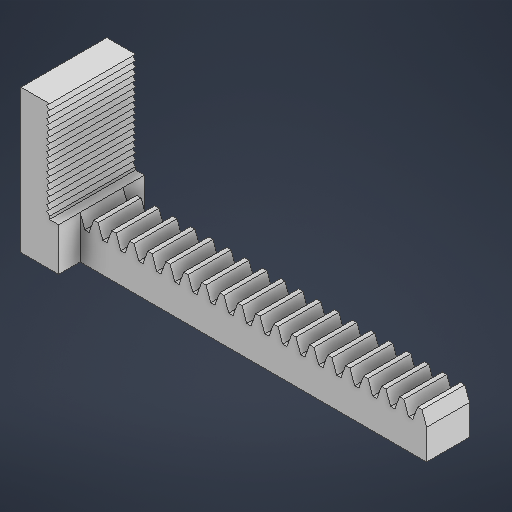
# Autodesk Inventor part: cremallera
Saved by Autodesk Inventor 2025.3 (Build 293356000, 356)
## iProperties
Created: 2024-05-21
Part Number: cremallera
Material: Genérico
Document SubType Name: Modeling
Designer: Jonathan Galarza
Density: 1 g/cm^3
Appearance: Valor por defecto
Author: Jonathan Galarza
Title: Cremallera
Autodesk Inventor part; units mm, degrees
ref_plane "YZ Plane" through (0, 0, 0) normal (1, 0, 0) x (0, 1, 0)
ref_plane "XZ Plane" through (0, 0, 0) normal (0, 1, 0) x (-1, 0, 0)
ref_plane "XY Plane" through (0, 0, 0) normal (0, 0, 1) x (1, 0, 0)
sketch "Boceto1" plane through (0, 0, 0) normal (0, 0, 1) x (1, 0, 0)
  line L0 (11.214, 2) -> (12.7381, 2)
  line L1 (9.5761, -2.5) -> (14.3759, -2.5)
  line L2 (10.486, 0) -> (7.5236, 0) construction
  line L3 (12.7381, 2) -> (14.3759, -2.5)
  line L4 (10.486, 0) -> (13.466, 0) construction
  line L5 (11.214, 2) -> (9.5761, -2.5)
  line L6 (13.466, 0) -> (10.486, 0) construction
  line L7 (17.494, 2) -> (19.0181, 2)
  line L8 (15.8561, -2.5) -> (20.6559, -2.5)
  line L9 (19.0181, 2) -> (20.6559, -2.5)
  line L10 (16.766, 0) -> (19.746, 0) construction
  line L11 (19.746, 0) -> (16.766, 0) construction
  line L12 (17.494, 2) -> (15.8561, -2.5)
  line L13 (23.774, 2) -> (25.2981, 2)
  line L14 (22.1361, -2.5) -> (26.9359, -2.5)
  line L15 (25.2981, 2) -> (26.9359, -2.5)
  line L16 (23.046, 0) -> (26.026, 0) construction
  line L17 (26.026, 0) -> (23.046, 0) construction
  line L18 (23.774, 2) -> (22.1361, -2.5)
  line L19 (30.054, 2) -> (31.5781, 2)
  line L20 (28.4161, -2.5) -> (33.2159, -2.5)
  line L21 (31.5781, 2) -> (33.2159, -2.5)
  line L22 (29.326, 0) -> (32.306, 0) construction
  line L23 (32.306, 0) -> (29.326, 0) construction
  line L24 (30.054, 2) -> (28.4161, -2.5)
  line L25 (36.334, 2) -> (37.8581, 2)
  line L26 (34.6961, -2.5) -> (39.4959, -2.5)
  line L27 (37.8581, 2) -> (39.4959, -2.5)
  line L28 (35.606, 0) -> (38.586, 0) construction
  line L29 (38.586, 0) -> (35.606, 0) construction
  line L30 (36.334, 2) -> (34.6961, -2.5)
  line L31 (42.614, 2) -> (44.1381, 2)
  line L32 (40.9761, -2.5) -> (45.7759, -2.5)
  line L33 (44.1381, 2) -> (45.7759, -2.5)
  line L34 (41.886, 0) -> (44.866, 0) construction
  line L35 (44.866, 0) -> (41.886, 0) construction
  line L36 (42.614, 2) -> (40.9761, -2.5)
  line L37 (48.894, 2) -> (50.4181, 2)
  line L38 (47.2561, -2.5) -> (52.0559, -2.5)
  line L39 (50.4181, 2) -> (52.0559, -2.5)
  line L40 (48.166, 0) -> (51.146, 0) construction
  line L41 (51.146, 0) -> (48.166, 0) construction
  line L42 (48.894, 2) -> (47.2561, -2.5)
  line L43 (55.174, 2) -> (56.6981, 2)
  line L44 (53.5361, -2.5) -> (58.3359, -2.5)
  line L45 (56.6981, 2) -> (58.3359, -2.5)
  line L46 (54.446, 0) -> (57.426, 0) construction
  line L47 (57.426, 0) -> (54.446, 0) construction
  line L48 (55.174, 2) -> (53.5361, -2.5)
  line L49 (61.454, 2) -> (62.9781, 2)
  line L50 (59.8161, -2.5) -> (64.6159, -2.5)
  line L51 (62.9781, 2) -> (64.6159, -2.5)
  line L52 (60.726, 0) -> (63.706, 0) construction
  line L53 (63.706, 0) -> (60.726, 0) construction
  line L54 (61.454, 2) -> (59.8161, -2.5)
  line L55 (67.734, 2) -> (69.2581, 2)
  line L56 (66.0961, -2.5) -> (70.8959, -2.5)
  line L57 (69.2581, 2) -> (70.8959, -2.5)
  line L58 (67.006, 0) -> (69.986, 0) construction
  line L59 (69.986, 0) -> (67.006, 0) construction
  line L60 (67.734, 2) -> (66.0961, -2.5)
  line L61 (74.014, 2) -> (75.5381, 2)
  line L62 (72.3761, -2.5) -> (77.1759, -2.5)
  line L63 (75.5381, 2) -> (77.1759, -2.5)
  line L64 (73.286, 0) -> (76.266, 0) construction
  line L65 (76.266, 0) -> (73.286, 0) construction
  line L66 (74.014, 2) -> (72.3761, -2.5)
  line L67 (80.294, 2) -> (81.8181, 2)
  line L68 (78.6561, -2.5) -> (83.4559, -2.5)
  line L69 (81.8181, 2) -> (83.4559, -2.5)
  line L70 (79.566, 0) -> (82.546, 0) construction
  line L71 (82.546, 0) -> (79.566, 0) construction
  line L72 (80.294, 2) -> (78.6561, -2.5)
  line L73 (86.574, 2) -> (88.0981, 2)
  line L74 (84.9361, -2.5) -> (89.7359, -2.5)
  line L75 (88.0981, 2) -> (89.7359, -2.5)
  line L76 (85.846, 0) -> (88.826, 0) construction
  line L77 (88.826, 0) -> (85.846, 0) construction
  line L78 (86.574, 2) -> (84.9361, -2.5)
  line L79 (92.854, 2) -> (94.3781, 2)
  line L80 (91.2161, -2.5) -> (96.0159, -2.5)
  line L81 (94.3781, 2) -> (96.0159, -2.5)
  line L82 (92.126, 0) -> (95.106, 0) construction
  line L83 (95.106, 0) -> (92.126, 0) construction
  line L84 (92.854, 2) -> (91.2161, -2.5)
  line L85 (99.134, 2) -> (100.6581, 2)
  line L86 (97.4961, -2.5) -> (102.2959, -2.5)
  line L87 (100.6581, 2) -> (102.2959, -2.5)
  line L88 (98.406, 0) -> (101.386, 0) construction
  line L89 (101.386, 0) -> (98.406, 0) construction
  line L90 (99.134, 2) -> (97.4961, -2.5)
  line L91 (105.414, 2) -> (106.9381, 2)
  line L92 (103.7761, -2.5) -> (108.5759, -2.5)
  line L93 (106.9381, 2) -> (108.5759, -2.5)
  line L94 (104.686, 0) -> (107.666, 0) construction
  line L95 (107.666, 0) -> (104.686, 0) construction
  line L96 (105.414, 2) -> (103.7761, -2.5)
  line L97 (111.694, 2) -> (113.2181, 2)
  line L98 (110.0561, -2.5) -> (114.8559, -2.5)
  line L99 (113.2181, 2) -> (114.8559, -2.5)
  line L100 (110.966, 0) -> (113.946, 0) construction
  line L101 (113.946, 0) -> (110.966, 0) construction
  line L102 (111.694, 2) -> (110.0561, -2.5)
  line L103 (117.974, 2) -> (119.4981, 2)
  line L104 (116.3361, -2.5) -> (121.1359, -2.5)
  line L105 (119.4981, 2) -> (121.1359, -2.5)
  line L106 (117.246, 0) -> (120.226, 0) construction
  line L107 (120.226, 0) -> (117.246, 0) construction
  line L108 (117.974, 2) -> (116.3361, -2.5)
  line L109 (124.254, 2) -> (125.7781, 2)
  line L110 (122.6161, -2.5) -> (127.4159, -2.5)
  line L111 (125.7781, 2) -> (127.4159, -2.5)
  line L112 (123.526, 0) -> (126.506, 0) construction
  line L113 (126.506, 0) -> (123.526, 0) construction
  line L114 (124.254, 2) -> (122.6161, -2.5)
  line L115 (130.534, 2) -> (132.0581, 2)
  line L116 (128.8961, -2.5) -> (133.6959, -2.5)
  line L117 (132.0581, 2) -> (133.6959, -2.5)
  line L118 (129.806, 0) -> (132.786, 0) construction
  line L119 (132.786, 0) -> (129.806, 0) construction
  line L120 (130.534, 2) -> (128.8961, -2.5)
  line L121 (9.5761, -2.5) -> (133.6959, -2.5)
  line L122 (133.6959, -2.5) -> (133.6959, -13)
  line L123 (133.6959, -13) -> (9.5761, -13)
  line L124 (9.5761, -13) -> (9.5761, -2.5)
  point P0 (0, 0)
  dimension "d5" = 2
  dimension "d6" = 2.5
  dimension "d7" = 70
  dimension "d8" = 2.98
  dimension "d11" = 6.28
  dimension "d18" = 10.5
  constraints: 248 end point, 40 point on line, 4 horizontal, 1 collinear, 1 parallel, 1 vertical, 268 other
  measures "d5" distance between parallel lines of L2 L0
  measures "d6" distance between parallel lines of L2 L1
  measures "d7" angle of L0 L3
  measures "d8" distance of L2.start L4.end
  measures "d11" distance of L0.start L7.start
extrude "Extrusión1" add sketch "Boceto1" along normal blind 15
sketch "Boceto2" plane through (9.5761, -13, 0) normal (-1, 0, 0) x (0, 0, 1)
  line L0 (0, 0) -> (15, 0) projected
  line L1 (7.5, 0) -> (22.5, 0)
  line L2 (22.5, 0) -> (22.5, 50)
  line L3 (22.5, 50) -> (-7.5, 50)
  line L4 (-7.5, 50) -> (-7.5, 0)
  line L5 (-7.5, 0) -> (7.5, 0)
  point P0 (0, 13)
  dimension "d19" = 15
  dimension "d20" = 50
  dimension "d21" = 30
  constraints: 10 end point, 3 perpendicular, 1 collinear, 1 midpoint, 1 vertical
  measures "d19" distance of L1.start L1.end
  measures "d20" distance of L1.end L2.end
  measures "d21" distance of L2.end L3.end
extrude "Extrusión2" add sketch "Boceto2" along normal blind 10
sketch "Boceto3" plane through (9.5761, -13, 22.5) normal (0, 0, 1) x (1, 0, 0)
  line L0 (0, 0) -> (0, 50) projected
  line L1 (0, 50) -> (-10, 50) projected
  line L2 (0, 50) -> (-1, 49)
  line L3 (-1, 49) -> (0, 48)
  line L4 (0, 50) -> (0, 48)
  point P0 (-9.5761, 13)
  constraints: 6 end point, 1 collinear, 1 perpendicular, 1 point on line
extrude "Extrusión3" cut sketch "Boceto3" against normal through all
pattern_linear "Patrón rectangular1" count 17 spacing 2 along (0, -1, 0) of "Extrusión3"
sketch "Boceto4" plane through (-0.4239, -13, 22.5) normal (0, 0, 1) x (1, 0, 0)
  line L0 (0, 0) -> (0, 50) projected
  line L1 (14.7999, 10.5) -> (13.162, 15) projected
  line L2 (0, 0) -> (13.162, 0)
  line L3 (13.162, 0) -> (13.162, 15)
  line L4 (13.162, 15) -> (0, 15)
  line L5 (0, 15) -> (0, 0)
  point P0 (0.4239, 13)
  point P1 (0, 15)
  constraints: 8 end point, 2 parallel, 1 horizontal, 1 perpendicular
extrude "Extrusión4" add sketch "Boceto4" against normal blind 30
